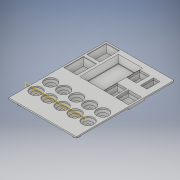
# Autodesk Inventor part: ds lite screw holder
Saved by Autodesk Inventor 2018.3 (Build 223284000, 284)
## iProperties
Created: 2019-06-14
Part Number: ds lite screw holder
Material: Generic
Document SubType Name: Modeling
Designer: Arjun Oberoi
Density: 1 g/cm^3
Appearance: Default
Author: Arjun Oberoi
Autodesk Inventor part; units mm, degrees
ref_plane "YZ Plane" through (0, 0, 0) normal (1, 0, 0) x (0, 1, 0)
ref_plane "XZ Plane" through (0, 0, 0) normal (0, 1, 0) x (-1, 0, 0)
ref_plane "XY Plane" through (0, 0, 0) normal (0, 0, 1) x (1, 0, 0)
sketch "Sketch1" plane through (0, 0, 0) normal (0, 1, 0) x (-1, 0, 0)
  circle A0 centre (38.1, 15.875) radius 11.43
  line L0 (0, 0) -> (13.476, 0) construction
  line L1 (0, 0) -> (0, -9.3151) construction
  circle A1 centre (12.7, 15.875) radius 11.43
  circle A2 centre (-12.7, 15.875) radius 11.43
  circle A3 centre (-38.1, 15.875) radius 11.43
  circle A4 centre (38.1, -12.7) radius 11.43
  circle A5 centre (12.7, -12.7) radius 11.43
  circle A6 centre (-12.7, -12.7) radius 11.43
  circle A7 centre (-38.1, -12.7) radius 11.43
  line L2 (50.165, -50.8) -> (24.765, -50.8)
  line L3 (24.765, -50.8) -> (24.765, -88.9)
  line L4 (24.765, -88.9) -> (50.165, -88.9)
  line L5 (50.165, -88.9) -> (50.165, -50.8)
  line L6 (12.065, -58.42) -> (-19.685, -58.42)
  line L7 (-19.685, -58.42) -> (-19.685, -118.745)
  line L8 (-19.685, -118.745) -> (12.065, -118.745)
  line L9 (12.065, -118.745) -> (12.065, -58.42)
  line L10 (53.34, 53.975) -> (-78.74, 53.975)
  line L11 (-78.74, 53.975) -> (-78.74, -136.525)
  line L12 (-78.74, -136.525) -> (53.34, -136.525)
  line L13 (53.34, -136.525) -> (53.34, 53.975)
  line L14 (24.765, -95.25) -> (24.765, -133.35)
  line L15 (24.765, -133.35) -> (50.165, -133.35)
  line L16 (50.165, -133.35) -> (50.165, -95.25)
  line L17 (50.165, -95.25) -> (24.765, -95.25)
  line L18 (-50.165, -50.8) -> (-75.565, -50.8)
  line L19 (-75.565, -50.8) -> (-75.565, -76.2)
  line L20 (-75.565, -76.2) -> (-50.165, -76.2)
  line L21 (-50.165, -76.2) -> (-50.165, -50.8)
  circle A8 centre (-63.5, 15.875) radius 11.43
  circle A9 centre (-63.5, -12.7) radius 11.43
  line L22 (-46.99, -50.8) -> (-27.94, -50.8)
  line L23 (-27.94, -50.8) -> (-27.94, -76.2)
  line L24 (-27.94, -76.2) -> (-46.99, -76.2)
  line L25 (-46.99, -76.2) -> (-46.99, -50.8)
  line L26 (-27.94, -120.65) -> (-46.99, -120.65)
  line L27 (-27.94, -95.25) -> (-27.94, -120.65)
  line L28 (-46.99, -95.25) -> (-27.94, -95.25)
  line L29 (-46.99, -120.65) -> (-46.99, -95.25)
  line L30 (-54.6227, -95.25) -> (-67.3227, -95.25)
  line L31 (-67.3227, -95.25) -> (-67.3227, -120.65)
  line L32 (-67.3227, -120.65) -> (-54.6227, -120.65)
  line L33 (-54.6227, -120.65) -> (-54.6227, -95.25)
  dimension "d0" = 22.86
  dimension "d3" = 25.4
  dimension "d6" = 28.575
  dimension "d9" = 12.7
  dimension "d10" = 12.7
  dimension "d11" = 25.4
  dimension "d12" = 38.1
  dimension "d20" = 38.1
  dimension "d21" = 31.75
  dimension "d22" = 60.325
  dimension "d23" = 38.1
  dimension "d24" = 15.24
  dimension "d47" = 44.45
  dimension "d52" = 3.175
  dimension "d53" = 3.175
  dimension "d54" = 12.7
  dimension "d55" = 25.4
  dimension "d56" = 25.4
  dimension "d57" = 3.175
  dimension "d58" = 30.48
  dimension "d59" = 15.24
  dimension "d85" = 7.62
  dimension "d114" = 19.05
  dimension "d115" = 25.4
  dimension "d116" = 3.175
  dimension "d130" = 44.45
  dimension "d141" = 12.7
  dimension "d142" = 25.4
  constraints: 68 end point, 12 parallel, 10 centre point, 8 horizontal, 6 perpendicular, 4 collinear, 4 vertical, 33 other
  measures "d0" diameter of A0
  measures "d3" distance of A0.centre A1.centre
  measures "d6" distance of A0.centre A4.centre
  measures "d9" distance from line of L1 A6.centre
  measures "d10" distance from line of L0 A5.centre
  measures "d11" distance of L4.end L3.end
  measures "d12" distance of L3.end L2.end
  measures "d20" distance from line of A4.centre L2
  measures "d21" distance of L8.end L7.end
  measures "d22" distance of L7.end L6.end
  measures "d23" distance from line of L10 A0.centre
  measures "d24" distance from line of A4.centre L13
  measures "d47" distance of L2.end L14.start
  measures "d52" distance between parallel lines of L12 L15
  measures "d53" distance between parallel lines of L13 L5
  measures "d54" distance between parallel lines of L3 L9
  measures "d55" distance of L20.end L19.end
  measures "d56" distance of L19.end L18.end
  measures "d57" distance between parallel lines of L11 L19
  measures "d58" distance between parallel lines of L7 L21
  measures "d59" distance from line of L11 A9.centre
  measures "d85" distance between parallel lines of L6 L18
  measures "d114" distance of L23.end L24.end
  measures "d115" distance of L22.end L23.end
  measures "d116" distance between parallel lines of L21 L25
  measures "d130" distance of L23.end L26.start
  measures "d141" distance of L32.end L31.end
  measures "d142" distance of L31.end L30.end
extrude "Extrusion1" add sketch "Sketch1" along normal blind 2.54
ref_plane "Work Plane2" through (-53.34, 0, 15.875) normal (0, 0, 1) x (1, 0, 0)
sketch "Sketch5" plane through (-53.34, 0, 15.875) normal (0, 0, 1) x (1, 0, 0)
  line L0 (80.01, 2.54) -> (102.87, 2.54) projected
  line L1 (102.87, 0) -> (80.01, 0) projected
  line L2 (77.47, 0) -> (54.61, 0) projected
  line L3 (80.01, 0) -> (85.09, -5.08)
  line L4 (85.09, -5.08) -> (91.44, -5.08)
  line L5 (102.87, 0) -> (80.01, 0) projected
  line L6 (91.44, -5.08) -> (91.44, 0) construction
  line L7 (102.87, 0) -> (80.01, 0) projected
  line L8 (77.47, 0) -> (85.09, -7.62)
  line L9 (85.09, -7.62) -> (91.44, -7.62)
  line L10 (77.47, 0) -> (77.47, 2.54) projected
  line L11 (91.44, -7.62) -> (91.44, -5.08)
  line L12 (77.47, 0) -> (80.01, 0)
  line L13 (132.08, 0) -> (0, 0) projected
  point P0 (53.34, 0)
  dimension "d32" = 11.43
  dimension "d33" = 5.08
  dimension "d34" = 2.54
  dimension "d35" = 2.54
  dimension "d36" = 45
  constraints: 14 end point, 2 parallel, 2 perpendicular, 1 horizontal, 1 midpoint, 1 other
  measures "d32" distance from line of L6 L1.end
  measures "d33" distance between parallel lines of L1 L4
  measures "d34" distance of L1.end L10.start
  measures "d35" distance between parallel lines of L4 L9
  measures "d36" angle of L1 L3
revolve "Revolution1" add sketch "Sketch5" angle 360 about axis through (38.1, -5.08, 15.875) along (0, 1, 0)
fillet "Fillet1" radius 6.35 1 edges at (44.45, -5.08, 15.875)
pattern_linear "Rectangular Pattern1" count 4 spacing 25.4 along (-1, 0, 0) count 2 spacing 28.575 along (0, 0, -1) of "Revolution1", "Fillet1"
pattern_linear "Rectangular Pattern2" count 2 spacing 25.4 along (1, 0, 0) of "Revolution1", "Fillet1", "Rectangular Pattern1"
sketch "Sketch7" plane through (0, 0, 0) normal (0, -1, 0) x (1, 0, 0)
  line L0 (78.74, -47.625) -> (46.99, -47.625)
  line L1 (46.99, -47.625) -> (46.99, -79.375)
  line L2 (46.99, -79.375) -> (78.74, -79.375)
  line L3 (78.74, -79.375) -> (78.74, -47.625)
  line L4 (78.74, 53.975) -> (78.74, -136.525) projected
  line L5 (75.565, -50.8) -> (75.565, -76.2) projected
  line L6 (50.165, -50.8) -> (75.565, -50.8) projected
  line L7 (50.165, -76.2) -> (50.165, -50.8) projected
  line L8 (75.565, -76.2) -> (50.165, -76.2) projected
  point P0 (0, 0)
  dimension "d63" = 3.175
  dimension "d64" = 3.175
  dimension "d65" = 3.175
  dimension "d66" = 3.175
  constraints: 8 end point, 2 parallel, 1 collinear, 1 horizontal, 1 perpendicular
  measures "d63" distance between parallel lines of L3 L5
  measures "d64" distance between parallel lines of L6 L0
  measures "d65" distance between parallel lines of L1 L7
  measures "d66" distance between parallel lines of L2 L8
extrude "Extrusion2" add sketch "Sketch7" along normal blind 7.62
sketch "Sketch8" plane through (0, -7.62, 0) normal (0, -1, 0) x (1, 0, 0)
  line L0 (46.99, -79.375) -> (78.74, -79.375) projected
  line L1 (46.99, -47.625) -> (46.99, -79.375) projected
  line L2 (78.74, -79.375) -> (46.99, -79.375)
  line L3 (46.99, -79.375) -> (46.99, -47.625)
  line L4 (46.99, -47.625) -> (78.74, -47.625)
  line L5 (78.74, -47.625) -> (78.74, -79.375)
  point P0 (0, 0)
  constraints: 8 end point, 2 parallel, 1 horizontal, 1 perpendicular
extrude "Extrusion3" add sketch "Sketch8" against normal blind 1.27
chamfer "Chamfer1" distance 3.175 angle 45 4 edges at (62.865, -6.35, -50.8) (75.565, -6.35, -63.5) (62.865, -6.35, -76.2) (50.165, -6.35, -63.5)
sketch "Sketch9" plane through (0, 0, 0) normal (0, -1, 0) x (1, 0, 0)
  line L0 (22.86, -121.92) -> (-15.24, -121.92)
  line L1 (-15.24, -121.92) -> (-15.24, -55.245)
  line L2 (-15.24, -55.245) -> (22.86, -55.245)
  line L3 (22.86, -55.245) -> (22.86, -121.92)
  line L4 (19.685, -118.745) -> (-12.065, -118.745) projected
  line L5 (-12.065, -118.745) -> (-12.065, -58.42) projected
  line L6 (19.685, -58.42) -> (19.685, -118.745) projected
  line L7 (-12.065, -58.42) -> (19.685, -58.42) projected
  point P0 (0, 0)
  dimension "d74" = 3.175
  dimension "d75" = 3.175
  dimension "d76" = 3.175
  dimension "d77" = 3.175
  constraints: 8 end point, 2 parallel, 1 horizontal, 1 perpendicular
  measures "d74" distance between parallel lines of L0 L4
  measures "d75" distance between parallel lines of L5 L1
  measures "d76" distance between parallel lines of L3 L6
  measures "d77" distance between parallel lines of L7 L2
extrude "Extrusion4" add sketch "Sketch9" along normal blind 7.62
sketch "Sketch10" plane through (0, -7.62, 0) normal (0, -1, 0) x (1, 0, 0)
  line L0 (22.86, -55.245) -> (-15.24, -55.245) projected
  line L1 (-15.24, -55.245) -> (-15.24, -121.92) projected
  line L2 (-15.24, -121.92) -> (22.86, -121.92) projected
  line L3 (22.86, -121.92) -> (22.86, -55.245) projected
  point P0 (0, 0)
extrude "Extrusion5" add sketch "Sketch10" against normal blind 1.27
chamfer "Chamfer2" distance 7.62 angle 45 8 edges at (3.81, 0, -121.92) (-15.24, 0, -88.5825) (3.81, 0, -55.245) (22.86, 0, -88.5825) (3.81, 2.54, -58.42) (-12.065, 2.54, -88.5825) (3.81, 2.54, -118.745) (19.685, 2.54, -88.5825)
sketch "Sketch11" plane through (0, 0, 0) normal (0, -1, 0) x (1, 0, 0)
  line L0 (-24.765, -50.8) -> (-24.765, -88.9) projected
  line L1 (-50.165, -50.8) -> (-24.765, -50.8) projected
  line L2 (-50.165, -88.9) -> (-50.165, -50.8) projected
  line L3 (-24.765, -88.9) -> (-50.165, -88.9) projected
  line L4 (-21.59, -47.625) -> (-53.34, -47.625)
  line L5 (-53.34, -47.625) -> (-53.34, -92.075)
  line L6 (-53.34, -92.075) -> (-21.59, -92.075)
  line L7 (-21.59, -92.075) -> (-21.59, -47.625)
  point P0 (0, 0)
  dimension "d86" = 3.175
  dimension "d87" = 3.175
  dimension "d88" = 3.175
  dimension "d89" = 3.175
  constraints: 8 end point, 2 parallel, 1 horizontal, 1 perpendicular
  measures "d86" distance between parallel lines of L0 L7
  measures "d87" distance between parallel lines of L1 L4
  measures "d88" distance between parallel lines of L3 L6
  measures "d89" distance between parallel lines of L2 L5
extrude "Extrusion6" add sketch "Sketch11" along normal blind 7.62
sketch "Sketch12" plane through (0, -7.62, 0) normal (0, -1, 0) x (1, 0, 0)
  line L0 (-24.765, -88.9) -> (-50.165, -88.9) projected
  line L1 (-50.165, -88.9) -> (-50.165, -50.8) projected
  line L2 (-50.165, -50.8) -> (-24.765, -50.8) projected
  line L3 (-24.765, -50.8) -> (-24.765, -88.9) projected
  line L4 (-21.59, -47.625) -> (-53.34, -47.625) projected
  line L5 (-53.34, -47.625) -> (-53.34, -92.075) projected
  line L6 (-53.34, -92.075) -> (-21.59, -92.075) projected
  line L7 (-21.59, -92.075) -> (-21.59, -47.625) projected
  point P0 (0, 0)
extrude "Extrusion7" add sketch "Sketch12" against normal blind 1.27 contours L0 L1 L2 L3
chamfer "Chamfer3" distance 7.62 angle 45 4 edges at (-50.165, -6.35, -69.85) (-37.465, -6.35, -88.9) (-24.765, -6.35, -69.85) (-37.465, -6.35, -50.8)
chamfer "Chamfer4" distance 5.08 angle 45 4 edges at (-21.59, -7.62, -69.85) (-37.465, -7.62, -92.075) (-53.34, -7.62, -69.85) (-37.465, -7.62, -47.625)
pattern_linear "Rectangular Pattern3" count 2 spacing 44.45 along (0, 0, -1) of "Extrusion7", "Extrusion6"
chamfer "Chamfer5" distance 7.62 angle 45 4 edges at (-50.165, -6.35, -114.3) (-37.465, -6.35, -133.35) (-24.765, -6.35, -114.3) (-37.465, -6.35, -95.25)
chamfer "Chamfer6" distance 5.08 angle 45 4 edges at (-37.465, -7.62, -92.075) (-53.34, -7.62, -114.3) (-37.465, -7.62, -136.525) (-21.59, -7.62, -114.3)
chamfer "Chamfer7" distance 5.08 angle 45 4 edges at (62.865, -7.62, -79.375) (46.99, -7.62, -63.5) (62.865, -7.62, -47.625) (78.74, -7.62, -63.5)
sketch "Sketch14" plane through (0, 0, 0) normal (0, -1, 0) x (1, 0, 0)
  line L0 (24.765, -47.625) -> (50.165, -47.625)
  line L1 (50.165, -47.625) -> (50.165, -79.375)
  line L2 (50.165, -79.375) -> (24.765, -79.375)
  line L3 (24.765, -79.375) -> (24.765, -47.625)
  line L4 (27.94, -50.8) -> (27.94, -76.2) projected
  line L5 (27.94, -50.8) -> (27.94, -76.2) projected
  line L6 (46.99, -50.8) -> (27.94, -50.8) projected
  line L7 (46.99, -76.2) -> (46.99, -50.8) projected
  line L8 (27.94, -76.2) -> (46.99, -76.2) projected
  point P0 (0, 0)
  dimension "d117" = 3.175
  dimension "d118" = 3.175
  dimension "d119" = 3.175
  dimension "d120" = 3.175
  constraints: 8 end point, 2 parallel, 1 horizontal, 1 perpendicular
  measures "d117" distance between parallel lines of L7 L1
  measures "d118" distance between parallel lines of L8 L2
  measures "d119" distance between parallel lines of L6 L0
  measures "d120" distance between parallel lines of L4 L3
extrude "Extrusion8" add sketch "Sketch14" along normal blind 7.62
sketch "Sketch16" plane through (0, -7.62, 0) normal (0, -1, 0) x (1, 0, 0)
  line L0 (46.99, -76.2) -> (27.94, -76.2) projected
  line L1 (27.94, -76.2) -> (27.94, -50.8) projected
  line L2 (27.94, -50.8) -> (46.99, -50.8) projected
  line L3 (46.99, -50.8) -> (46.99, -76.2) projected
  line L4 (50.165, -47.625) -> (24.765, -47.625) projected
  line L5 (24.765, -47.625) -> (24.765, -79.375) projected
  line L6 (24.765, -79.375) -> (50.165, -79.375) projected
  line L7 (50.165, -79.375) -> (50.165, -47.625) projected
  point P0 (0, 0)
extrude "Extrusion9" add sketch "Sketch16" against normal blind 1.27 contours L0 L1 L2 L3
chamfer "Chamfer8" distance 5.08 angle 45 4 edges at (27.94, -6.35, -63.5) (37.465, -6.35, -50.8) (46.99, -6.35, -63.5) (37.465, -6.35, -76.2)
pattern_linear "Rectangular Pattern4" count 2 spacing 44.45 along (0, 0, -1) of "Extrusion8", "Extrusion9"
chamfer "Chamfer9" distance 5.08 angle 45 4 edges at (27.94, -6.35, -107.95) (37.465, -6.35, -95.25) (46.99, -6.35, -107.95) (37.465, -6.35, -120.65)
sketch "Sketch18" plane through (0, 0, 0) normal (0, -1, 0) x (1, 0, 0)
  line L0 (70.4977, -92.075) -> (51.4477, -92.075)
  line L1 (51.4477, -92.075) -> (51.4477, -123.825)
  line L2 (51.4477, -123.825) -> (70.4977, -123.825)
  line L3 (70.4977, -123.825) -> (70.4977, -92.075)
  line L4 (54.6227, -120.65) -> (54.6227, -95.25) projected
  line L5 (67.3227, -120.65) -> (54.6227, -120.65) projected
  line L6 (67.3227, -95.25) -> (67.3227, -120.65) projected
  line L7 (54.6227, -95.25) -> (67.3227, -95.25) projected
  point P0 (0, 0)
  dimension "d143" = 3.175
  dimension "d144" = 3.175
  dimension "d145" = 3.175
  dimension "d146" = 3.175
  constraints: 8 end point, 2 parallel, 1 horizontal, 1 perpendicular
  measures "d143" distance between parallel lines of L1 L4
  measures "d144" distance between parallel lines of L5 L2
  measures "d145" distance between parallel lines of L6 L3
  measures "d146" distance between parallel lines of L7 L0
extrude "Extrusion10" add sketch "Sketch18" along normal blind 7.62
sketch "Sketch19" plane through (0, -7.62, 0) normal (0, -1, 0) x (1, 0, 0)
  line L0 (54.6227, -95.25) -> (67.3227, -95.25) projected
  line L1 (67.3227, -95.25) -> (67.3227, -120.65) projected
  line L2 (67.3227, -120.65) -> (54.6227, -120.65) projected
  line L3 (54.6227, -120.65) -> (54.6227, -95.25) projected
  line L4 (70.4977, -92.075) -> (51.4477, -92.075) projected
  line L5 (51.4477, -92.075) -> (51.4477, -123.825) projected
  line L6 (51.4477, -123.825) -> (70.4977, -123.825) projected
  line L7 (70.4977, -123.825) -> (70.4977, -92.075) projected
  point P0 (0, 0)
extrude "Extrusion11" add sketch "Sketch19" against normal blind 1.27 contours L0 L1 L2 L3
chamfer "Chamfer10" distance 5.08 angle 45 4 edges at (54.6227, -6.35, -107.95) (60.9727, -6.35, -95.25) (67.3227, -6.35, -107.95) (60.9727, -6.35, -120.65)
sketch "Sketch20" plane through (0, 0, 0) normal (0, -1, 0) x (1, 0, 0)
  circle A0 centre (-40.64, 41.275) radius 6.35
  line L0 (-53.34, -47.625) -> (-53.34, 53.975) projected
  line L1 (-53.34, 53.975) -> (78.74, 53.975) projected
  circle A1 centre (66.04, 41.275) radius 6.35
  line L2 (78.74, 53.975) -> (78.74, -47.625) projected
  point P0 (0, 0)
  dimension "d154" = 12.7
  dimension "d155" = 12.7
  dimension "d156" = 12.7
  dimension "d157" = 12.7
  dimension "d158" = 12.7
  dimension "d159" = 12.7
  constraints: 2 centre point
  measures "d154" diameter of A0
  measures "d155" distance from line of L0 A0.centre
  measures "d156" distance from line of L1 A0.centre
  measures "d157" diameter of A1
  measures "d158" distance from line of L2 A1.centre
  measures "d159" distance from line of L1 A1.centre
extrude "Extrusion12" add sketch "Sketch20" along normal blind 7.62
equation "\"d35\" = d34"
equation "\"d64\" = d63"
equation "\"d65\" = d63"
equation "\"d66\" = d63"
body "Solid1"
